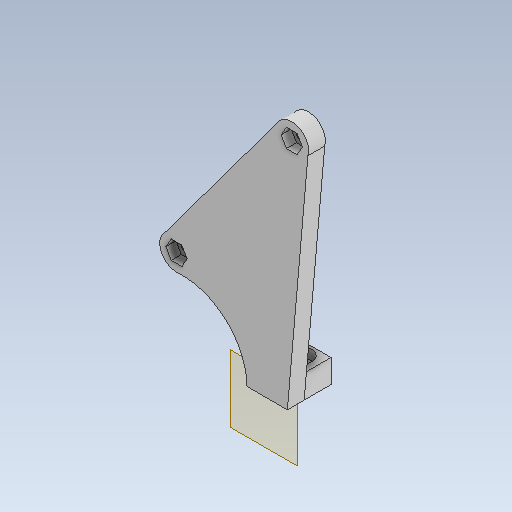
# Autodesk Inventor part: Fan Support Rear Left V2
Saved by Autodesk Inventor 2020 (Build 240168000, 168)
## iProperties
Created: 2019-12-06
Part Number: Fan Support Rear Left V2
Material: Generic
Document SubType Name: Modeling
Designer: pepd9
Density: 1 g/cm^3
Appearance: Default
Author: pepd9
Autodesk Inventor part; units mm, degrees
ref_plane "YZ Plane" through (0, 0, 0) normal (1, 0, 0) x (0, 1, 0)
ref_plane "XZ Plane" through (0, 0, 0) normal (0, 1, 0) x (-1, 0, 0)
ref_plane "Work Plane1" through (0, 0, 0.4) normal (0, 0, 1) x (1, 0, 0)
sketch "Sketch1" plane through (0, 0, 0.4) normal (0, 0, 1) x (1, 0, 0)
  circle A0 centre (-21, 32) radius 1.3
  circle A1 centre (13.3199, 77.9907) radius 5
  line L0 (0, 8) -> (12, 8)
  circle A2 centre (-5.1038, 53.7097) radius 15.8
  line L1 (12, 8) -> (18.1186, 76.5861)
  circle A3 centre (-21, 32) radius 5
  arc A4 (0, 8) -> (-21, 27) centre (-19.3877, 7.6767) ccw
  line L2 (8.9163, 80.3588) -> (-24.1358, 35.8944)
  point P0 (0, 0)
  dimension "d1" = 32
  dimension "d2" = 21
  dimension "d5" = 77.9907
  dimension "d6" = 13.32
  dimension "d7" = 8
  dimension "d8" = 10
  dimension "d9" = 10
  constraints: 6 end point, 6 point on circle, 5 centre point, 1 coincident
  measures "d1" vertical distance of point (0, 0) A0.centre
  measures "d2" horizontal distance of A0.centre point (0, 0)
  measures "d5" vertical distance of point (0, 0) A1.centre
  measures "d6" horizontal distance of point (0, 0) A1.centre
  measures "d7" distance from line of point (0, 0) L0
  measures "d8" diameter of A1
  measures "d9" diameter of A3
extrude "Extrusion1" add sketch "Sketch1" along normal blind 5 contours A0 | A1 | A1 L1 L0 A4 A3 L2 A2 | A2 L2 | A3 A4 picked at (-1.3107, 48.2112) picked at (-17.2977, 32.5158)
sketch "Sketch2" plane through (0, 0, 0.4) normal (0, 0, -1) x (-1, 0, 0)
  arc A0 (21, 27) -> (0, 8) centre (19.3877, 7.6767) ccw projected
  arc A1 (21, 27) -> (24.1358, 35.8944) centre (21, 32) ccw projected
  line L0 (-8.9163, 80.3588) -> (24.1358, 35.8944) projected
  arc A2 (-8.9163, 80.3588) -> (-18.1186, 76.5861) centre (-13.3199, 77.9907) ccw projected
  line L1 (-12, 8) -> (-18.1186, 76.5861) projected
  line L2 (0, 8) -> (-12, 8) projected
  line L3 (0, 8) -> (-12, 8) projected
  line L4 (-12, 8) -> (0, 8)
  line L5 (0, 8) -> (0, 15)
  line L6 (0, 15) -> (-12, 15)
  line L7 (-12, 15) -> (-12, 8)
  point P0 (0, 0)
  dimension "d12" = 7
  constraints: 8 end point, 2 parallel, 1 horizontal, 1 perpendicular
  measures "d12" distance of L5.end L4.end
extrude "Extrusion2" add sketch "Sketch2" along normal blind 8 contours L2 L7 L6 L5
sketch "Sketch3" plane through (0, 8, 5.4) normal (0, -1, 0) x (1, 0, 0)
  line L0 (3, -6.4) -> (1.8, -6.4) projected
  line L1 (3, -11.4) -> (3, -6.4) projected
  line L2 (1.8, -11.4) -> (3, -11.4) projected
  line L3 (1.8, -6.4) -> (1.8, -11.4) projected
  point P0 (0, -5.4)
extrude "Extrusion3" add sketch "Sketch3" along normal blind 2
sketch "Sketch4" plane through (0, 15, 0.4) normal (0, 1, 0) x (1, 0, 0)
  line L0 (0, 8) -> (12, 8) projected
  line L1 (12, 0) -> (12, 8) projected
  point P0 (0, 0.4)
  point P1 (7, 4)
  dimension "d17" = 4
  dimension "d18" = 5
  measures "d17" distance from line of L0 point (7, 4)
  measures "d18" distance from line of L1 point (7, 4)
hole "Hole1" at (7, 15, -3.6) direction (0, -1, 0) diameter 3.4 end through all counterbore diameter 6.5 counterbore depth 3 clearance for "Socket Head Cap Screw" size "M3" standard "Ansi Metric M Profile"
sketch "Sketch5" plane through (0, 0, 5.4) normal (0, 0, 1) x (1, 0, 0)
  arc A0 (-24.1358, 35.8944) -> (-21, 27) centre (-21, 32) ccw projected
  arc A1 (18.1186, 76.5861) -> (8.9163, 80.3588) centre (13.3199, 77.9907) ccw projected
  point P0 (0, 0)
hole "Hole2" at (-21, 32, 5.4) at (13.3199, 77.9907, 5.4) direction (0, 0, -1) diameter 3.4 end through all clearance for "Socket Head Cap Screw" size "M3" standard "Ansi Metric M Profile"
sketch "Sketch6" plane through (0, 0, 5.4) normal (0, 0, 1) x (1, 0, 0)
  circle A0 centre (-21, 32) radius 1.7 projected
  circle A1 centre (13.3199, 77.9907) radius 1.7 projected
  line L0 (-19.4123, 34.75) -> (-17.8246, 32)
  line L1 (-17.8246, 32) -> (-19.4123, 29.25)
  line L2 (-19.4123, 29.25) -> (-22.5877, 29.25)
  line L3 (-22.5877, 29.25) -> (-24.1754, 32)
  line L4 (-24.1754, 32) -> (-22.5877, 34.75)
  line L5 (-22.5877, 34.75) -> (-19.4123, 34.75)
  line L6 (11.7322, 75.2407) -> (10.1445, 77.9907)
  line L7 (10.1445, 77.9907) -> (11.7322, 80.7407)
  line L8 (11.7322, 80.7407) -> (14.9077, 80.7407)
  line L9 (14.9077, 80.7407) -> (16.4954, 77.9907)
  line L10 (16.4954, 77.9907) -> (14.9077, 75.2407)
  line L11 (14.9077, 75.2407) -> (11.7322, 75.2407)
  point P0 (0, 0)
  dimension "d33" = 5.5
  dimension "d34" = 5.5
  constraints: 24 end point, 2 coincident, 2 horizontal, 26 other
  measures "d33" distance between parallel lines of L5 L2
  measures "d34" distance between parallel lines of L11 L8
extrude "Extrusion4" cut sketch "Sketch6" against normal blind 3 contours A0 | A1 | L0 L1 L2 L3 L4 L5 | L6 L7 L8 L9 L10 L11
body "Solid1"
